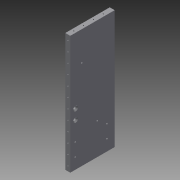
# Autodesk Inventor part: Yagi_BaseFrame
Saved by Autodesk Inventor 2014 (Build 180170000, 170)
## iProperties
Created: 2015-01-07
Part Number: Yagi_BaseFrame
Material: Generic
Document SubType Name: Modeling
Designer: Owner
Density: 1 g/cm^3
Appearance: Default
Author: Owner
Autodesk Inventor part; units mm, degrees
ref_plane "YZ Plane" through (0, 0, 0) normal (1, 0, 0) x (0, 1, 0)
ref_plane "XZ Plane" through (0, 0, 0) normal (0, 1, 0) x (-1, 0, 0)
ref_plane "XY Plane" through (0, 0, 0) normal (0, 0, 1) x (1, 0, 0)
sketch "Sketch1" plane through (0, 0, 0) normal (0, 0, 1) x (1, 0, 0)
  line L0 (65.2483, 137.2649) -> (65.2483, -15.1351)
  line L1 (71.5983, 137.2649) -> (71.5983, -15.1351)
  line L2 (65.2483, -15.1351) -> (71.5983, -15.1351)
  line L3 (65.2483, 137.2649) -> (71.5983, 137.2649)
  line L4 (65.2483, 128.3749) -> (65.2483, 131.5499)
  line L5 (65.2483, 47.6029) -> (65.2483, 44.4279)
  point P0 (0, 0)
  dimension "d1" = 152.4
  dimension "d21" = 6.35
  constraints: 12 end point, 2 point on line, 1 horizontal, 1 parallel, 1 perpendicular
  measures "d1" distance of L0.start L0.end
  measures "d21" distance of L0.start L1.start
extrude "Extrusion1" add sketch "Sketch1" along normal blind 57.15
sketch "Sketch2" plane through (71.5983, -15.1351, 0) normal (1, 0, 0) x (0, 0, -1)
  point P0 (-50.175, 67.9)
hole "Hole1" at (71.5983, 52.7649, 50.175) direction (-1, 0, 0) diameter 3.4544 depth 6.35 countersink diameter 6.4008 countersink angle 82
pattern_linear "Rectangular Pattern1" count 2 spacing 12.7 along (0, -1, 0) of "Hole1"
sketch "Sketch5" plane through (65.2483, 137.2649, 0) normal (0, 1, 0) x (1, 0, 0)
  point P0 (3.175, -49.53)
hole "Hole6" at (68.4233, 137.2649, 49.53) direction (0, -1, 0) diameter 1.1811 depth 4.699 tip angle 120 thread size "0-80 UNF" class "2B" standard "ANSI Unified Screw Threads"
pattern_linear "Rectangular Pattern3" count 4 spacing 12.7 along (0, 0, -1) of "Hole6"
sketch "Sketch6" plane through (65.2483, -15.1351, 0) normal (0, -1, 0) x (1, 0, 0)
  point P0 (3.175, 49.53)
hole "Hole8" at (68.4233, -15.1351, 49.53) direction (0, 1, 0) diameter 1.1811 depth 4.699 tip angle 120 thread size "0-80 UNF" class "2B" standard "ANSI Unified Screw Threads"
pattern_linear "Rectangular Pattern4" count 4 spacing 12.7 along (0, 0, -1) of "Hole8"
sketch "Sketch7" plane through (71.5983, -15.1351, 0) normal (1, 0, 0) x (0, 0, -1)
  point P0 (-22.3759, 40.639)
hole "Hole10" at (71.5983, 25.5039, 22.3759) direction (-1, 0, 0) diameter 1.778 depth 6.35
sketch "Sketch8" plane through (71.5983, -15.1351, 0) normal (1, 0, 0) x (0, 0, -1)
  point P0 (-9.8029, 31.114)
hole "Hole12" at (71.5983, 15.9789, 9.8029) direction (-1, 0, 0) diameter 1.778 depth 6.35
sketch "Sketch9" plane through (71.5983, -15.1351, 0) normal (1, 0, 0) x (0, 0, -1)
  point P0 (-9.8029, 14.35)
hole "Hole14" at (71.5983, -0.7851, 9.8029) direction (-1, 0, 0) diameter 1.778 depth 6.35
sketch "Sketch10" plane through (71.5983, -15.1351, 0) normal (1, 0, 0) x (0, 0, -1)
  point P0 (-50.6969, 31.114)
hole "Hole16" at (71.5983, 15.9789, 50.6969) direction (-1, 0, 0) diameter 1.778 depth 6.35
sketch "Sketch11" plane through (71.5983, -15.1351, 0) normal (1, 0, 0) x (0, 0, -1)
  point P0 (-50.6969, 14.35)
hole "Hole18" at (71.5983, -0.7851, 50.6969) direction (-1, 0, 0) diameter 1.778 depth 6.35
sketch "Sketch12" plane through (71.5983, -15.1351, 0) normal (1, 0, 0) x (0, 0, -1)
  point P0 (-42.1244, 114.934)
hole "Hole20" at (71.5983, 99.7989, 42.1244) direction (-1, 0, 0) diameter 1.778 depth 6.35
sketch "Sketch13" plane through (0, 0, 0) normal (0, 0, -1) x (-1, 0, 0)
  point P0 (-68.4233, 130.9149)
hole "Hole22" at (68.4233, 130.9149, 0) direction (0, 0, 1) diameter 1.778 depth 57.15
pattern_linear "Rectangular Pattern5" count 12 spacing 12.7 along (0, -1, 0) of "Hole22"
body "Solid1"
